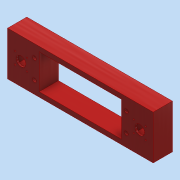
# Autodesk Inventor part: antennae_holder
Saved by Autodesk Inventor 2022 (Build 260153000, 153)
## iProperties
Created: 2020-03-02
Part Number: antennae_holder
Material: Generic
Document SubType Name: Modeling
Designer: nnico
Density: 1 g/cm^3
Appearance: Red
Author: nnico
Autodesk Inventor part; units mm, degrees
ref_plane "YZ Plane" through (0, 0, 0) normal (1, 0, 0) x (0, 1, 0)
ref_plane "XZ Plane" through (0, 0, 0) normal (0, 1, 0) x (-1, 0, 0)
ref_plane "XY Plane" through (0, 0, 0) normal (0, 0, 1) x (1, 0, 0)
sketch "Sketch1" plane through (0, 0, 0) normal (0, 1, 0) x (-1, 0, 0)
  line L0 (190, -57.5) -> (-190, -57.5)
  line L1 (-190, -57.5) -> (-190, 57.5)
  line L2 (-190, 57.5) -> (190, 57.5)
  line L3 (190, 57.5) -> (190, -57.5)
  line L4 (0, -57.5) -> (0, 57.5) construction
  line L5 (190, 0) -> (-190, 0) construction
  point P0 (0, 0)
  point P1 (0, 0)
  dimension "d0" = 380
  dimension "d1" = 115
  constraints: 12 end point, 5 midpoint, 2 parallel, 1 coincident, 1 horizontal, 1 perpendicular
  measures "d0" distance of L0.start L0.end
  measures "d1" distance of L2.end L0.start
extrude "Extrusion1" add sketch "Sketch1" along normal blind 50
sketch "Sketch2" plane through (0, 50, 0) normal (0, 1, 0) x (1, 0, 0)
  line L0 (-177.5, 22.5) -> (-132.5, 22.5)
  line L1 (-132.5, 22.5) -> (-132.5, -22.5)
  line L2 (-132.5, -22.5) -> (-177.5, -22.5)
  line L3 (-177.5, -22.5) -> (-177.5, 22.5)
  line L4 (190, 57.5) -> (-190, 57.5) construction
  line L5 (0, 57.5) -> (0, -57.5) construction
  line L6 (-190, -57.5) -> (190, -57.5) construction
  line L7 (-190, 57.5) -> (-190, -57.5) construction
  line L8 (-190, 0) -> (190, 0) construction
  line L9 (190, -57.5) -> (190, 57.5) construction
  line L10 (-177.5, 0) -> (-132.5, 0) construction
  line L11 (-155, 22.5) -> (-155, -22.5) construction
  line L12 (177.5, 22.5) -> (132.5, 22.5)
  line L13 (132.5, 22.5) -> (132.5, -22.5)
  line L14 (132.5, -22.5) -> (177.5, -22.5)
  line L15 (177.5, -22.5) -> (177.5, 22.5)
  point P0 (0, 0)
  dimension "d4" = 45
  dimension "d5" = 45
  dimension "d6" = 310
  constraints: 24 end point, 8 midpoint, 4 symmetric about line, 2 parallel, 1 collinear, 1 horizontal, 1 perpendicular
  measures "d4" distance of L1.end L2.end
  measures "d5" distance of L0.end L1.end
  measures "d6" diameter of L11.start L5
extrude "Extrusion2" cut sketch "Sketch2" against normal blind 45
sketch "Sketch3" plane through (0, 50, 0) normal (0, 1, 0) x (1, 0, 0)
  line L0 (190, 57.5) -> (-190, 57.5) construction
  line L1 (0, 57.5) -> (0, -57.5) construction
  line L2 (-190, -57.5) -> (190, -57.5) construction
  line L3 (-132.5, 22.5) -> (-132.5, -22.5) construction
  line L4 (-132.5, 0) -> (132.5, 0) construction
  line L5 (132.5, -22.5) -> (132.5, 22.5) construction
  line L6 (-120, 25) -> (-120, -25) construction
  circle A0 centre (-120, 25) radius 2.5
  circle A1 centre (-120, -25) radius 2.25
  circle A2 centre (120, 25) radius 2.5
  circle A3 centre (120, -25) radius 2.25
  point P0 (0, 0)
  dimension "d15" = 50
  dimension "d16" = 5
  dimension "d17" = 4.5
  dimension "d18" = 50
  dimension "d19" = 240
  constraints: 6 end point, 4 centre point, 4 coincident, 4 midpoint, 4 symmetric about line, 1 perpendicular, 2 other
  measures "d15" distance of L6.start L6.end
  measures "d16" diameter of A0
  measures "d17" diameter of A1
  measures "d18" diameter of L6.start L4
  measures "d19" diameter of L6.start L1
extrude "Extrusion3" cut sketch "Sketch3" against normal up to next
sketch "Sketch4" plane through (0, 50, 0) normal (0, 1, 0) x (1, 0, 0)
  line L0 (107.5, -45) -> (-107.5, -45)
  line L1 (-107.5, -45) -> (-107.5, 45)
  line L2 (-107.5, 45) -> (107.5, 45)
  line L3 (107.5, 45) -> (107.5, -45)
  line L4 (0, -45) -> (0, 45) construction
  line L5 (107.5, 0) -> (-107.5, 0) construction
  circle A0 centre (120, -25) radius 2.25 projected
  point P0 (0, 0)
  point P1 (0, 0)
  dimension "d23" = 90
  dimension "d29" = 12.5
  constraints: 12 end point, 5 midpoint, 2 parallel, 1 coincident, 1 horizontal, 1 perpendicular
  measures "d23" distance of L0.end L1.end
  measures "d29" distance from line of L3 A0.centre
extrude "Extrusion4" cut sketch "Sketch4" against normal up to next contours L0 L1 L2 L3
sketch "Sketch5" plane through (0, 5, 0) normal (0, 1, 0) x (1, 0, 0)
  line L0 (-190, -57.5) -> (190, -57.5) construction
  line L1 (0, -57.5) -> (0, 57.5) construction
  line L2 (190, 57.5) -> (-190, 57.5) construction
  line L3 (132.5, -22.5) -> (132.5, 22.5) construction
  line L4 (177.5, -22.5) -> (132.5, -22.5) construction
  line L5 (177.5, 22.5) -> (177.5, -22.5) construction
  line L6 (132.5, 22.5) -> (177.5, 22.5) construction
  line L7 (177.5, -22.5) -> (132.5, -22.5) construction
  line L8 (155, -22.5) -> (155, 22.5) construction
  line L9 (132.5, 22.5) -> (177.5, 22.5) construction
  line L10 (177.5, 22.5) -> (177.5, -22.5) construction
  line L11 (177.5, 0) -> (132.5, 0) construction
  line L12 (132.5, -22.5) -> (132.5, 22.5) construction
  circle A0 centre (155, 0) radius 12.5
  circle A1 centre (-155, 0) radius 12.5
  point P0 (0, 0)
  dimension "d26" = 25
  constraints: 7 midpoint, 6 end point, 2 centre point, 1 symmetric about line, 1 other
  measures "d26" diameter of A0
extrude "Extrusion5" cut sketch "Sketch5" against normal up to next
sketch "Sketch6" plane through (0, 5, 0) normal (0, 1, 0) x (1, 0, 0)
  line L0 (190, 57.5) -> (-190, 57.5) construction
  line L1 (0, 57.5) -> (0, -57.5) construction
  line L2 (190, -57.5) -> (-190, -57.5) construction
  line L3 (-170.5, 15.5) -> (-139.5, 15.5) construction
  line L4 (-139.5, 15.5) -> (-139.5, -15.5) construction
  line L5 (-139.5, -15.5) -> (-170.5, -15.5) construction
  line L6 (-170.5, -15.5) -> (-170.5, 15.5) construction
  line L7 (-177.5, 22.5) -> (-132.5, 22.5) construction
  line L8 (-132.5, -22.5) -> (-177.5, -22.5) construction
  line L9 (-155, 22.5) -> (-155, -22.5) construction
  line L10 (-177.5, -22.5) -> (-177.5, 22.5) construction
  line L11 (-177.5, 0) -> (-132.5, 0) construction
  line L12 (-132.5, 22.5) -> (-132.5, -22.5) construction
  line L13 (-170.5, 0) -> (-139.5, 0) construction
  line L14 (-155, -15.5) -> (-155, 15.5) construction
  circle A0 centre (-170.5, 15.5) radius 1.75
  circle A1 centre (-139.5, 15.5) radius 1.5
  circle A2 centre (-170.5, -15.5) radius 1.5
  circle A3 centre (-139.5, -15.5) radius 1.5
  circle A4 centre (170.5, 15.5) radius 1.75
  circle A5 centre (139.5, 15.5) radius 1.5
  circle A6 centre (170.5, -15.5) radius 1.5
  circle A7 centre (139.5, -15.5) radius 1.5
  point P0 (0, 0)
  point P1 (-155, 0)
  dimension "d30" = 31
  dimension "d31" = 31
  dimension "d32" = 3.5
  dimension "d33" = 3
  dimension "d34" = 3
  dimension "d35" = 3
  constraints: 18 end point, 12 midpoint, 8 centre point, 4 coincident, 4 symmetric about line, 2 parallel, 1 horizontal, 1 perpendicular, 4 other
  measures "d30" distance of L4.end L5.end
  measures "d31" distance of L3.end L4.end
  measures "d32" diameter of A0
  measures "d33" diameter of A1
  measures "d34" diameter of A2
  measures "d35" diameter of A3
extrude "Extrusion6" cut sketch "Sketch6" against normal up to next
sketch "Sketch7" plane through (0, 50, 0) normal (0, 1, 0) x (1, 0, 0)
  line L0 (-190, 57.5) -> (190, 57.5) construction
  line L1 (0, 57.5) -> (0, -57.5) construction
  line L2 (190, -57.5) -> (-190, -57.5) construction
  line L3 (-177.5, 22.5) -> (-132.5, 22.5) projected
  line L4 (-160, 22.5) -> (-150, 22.5)
  line L5 (-150, 22.5) -> (-150, 27.5)
  line L6 (-150, 27.5) -> (-160, 27.5)
  line L7 (-160, 27.5) -> (-160, 22.5)
  line L8 (-155, 27.5) -> (-155, 22.5) construction
  line L9 (160, 22.5) -> (150, 22.5)
  line L10 (150, 22.5) -> (150, 27.5)
  line L11 (150, 27.5) -> (160, 27.5)
  line L12 (160, 27.5) -> (160, 22.5)
  point P0 (0, 0)
  dimension "d38" = 10
  dimension "d39" = 5
  dimension "d40" = 22.5
  constraints: 20 end point, 4 midpoint, 4 symmetric about line, 2 parallel, 1 horizontal, 1 perpendicular, 1 point on line
  measures "d38" distance of L6.end L5.end
  measures "d39" distance of L5.end L4.end
  measures "d40" distance of L3.start L8.end
extrude "Extrusion7" cut sketch "Sketch7" against normal blind 45
sketch "Sketch8" plane through (0, 0, 0) normal (0, -1, 0) x (1, 0, 0)
  circle A0 centre (-120, 25) radius 2.25 projected
  circle A1 centre (-120, 25) radius 5
  line L0 (-190, -57.5) -> (-190, 57.5) construction
  line L1 (-190, 0) -> (190, 0) construction
  line L2 (190, 57.5) -> (190, -57.5) construction
  line L3 (-190, -57.5) -> (190, -57.5) construction
  line L4 (0, -57.5) -> (0, 57.5) construction
  line L5 (190, 57.5) -> (-190, 57.5) construction
  circle A2 centre (-120, -25) radius 5
  circle A3 centre (120, 25) radius 5
  circle A4 centre (120, -25) radius 5
  point P0 (0, 0)
  dimension "d43" = 10
  constraints: 4 centre point, 4 end point, 4 midpoint, 3 symmetric about line, 1 coincident, 3 other
  measures "d43" diameter of A1
extrude "Extrusion8" cut sketch "Sketch8" against normal blind 40
body "Solid1"
